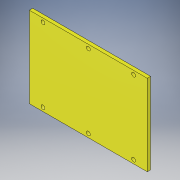
# Autodesk Inventor part: КВ33.000.104 - Крышка
Saved by Autodesk Inventor 2019 (Build 230136000, 136)
## iProperties
Created: 2021-03-13
Part Number: КВ33.000.104 - Крышка
Material: ABS Plastic
Document SubType Name: Modeling
Designer: Петров Иван
Density: 1.06 g/cm^3
Appearance: Yellow
Author: Петров Иван
Autodesk Inventor part; units mm, degrees
ref_plane "YZ Plane" through (0, 0, 0) normal (1, 0, 0) x (0, 1, 0)
ref_plane "XZ Plane" through (0, 0, 0) normal (0, 1, 0) x (-1, 0, 0)
ref_plane "XY Plane" through (0, 0, 0) normal (0, 0, 1) x (1, 0, 0)
sketch "Sketch1" plane through (0, 0, 0) normal (0, 0, 1) x (1, 0, 0)
  circle A0 centre (40, -0.1123) radius 1.75 projected
  circle A1 centre (0, -0.1123) radius 1.75 projected
  circle A2 centre (-40, -0.1123) radius 1.75 projected
  line L0 (-44, 3.3877) -> (44, 3.3877) projected
  line L1 (-44, -3.3877) -> (-44, 3.3877) projected
  line L2 (44, -3.3877) -> (-44, -3.3877) projected
  line L3 (44, 3.3877) -> (44, -3.3877) projected
  circle A3 centre (-40, 64.7863) radius 1.75 projected
  circle A4 centre (0, 64.7863) radius 1.75 projected
  circle A5 centre (40, 64.7863) radius 1.75 projected
  line L4 (44, 61.2863) -> (-44, 61.2863) projected
  line L5 (44, 68.0616) -> (44, 61.2863) projected
  line L6 (-44, 68.0616) -> (44, 68.0616) projected
  line L7 (-44, 61.2863) -> (-44, 68.0616) projected
  line L8 (44, 68.0616) -> (44, -3.3877) projected
  line L9 (44, -3.3877) -> (47, -3.3877) projected
  line L10 (47, 68.0616) -> (47, -3.3877) projected
  line L11 (44, 68.0616) -> (47, 68.0616) projected
  line L12 (-47, 68.0616) -> (-47, -3.3877) projected
  line L13 (-47, -3.3877) -> (-44, -3.3877) projected
  line L14 (-44, 68.0616) -> (-44, -3.3877) projected
  line L15 (-47, 68.0616) -> (-44, 68.0616) projected
  line L16 (-47, -3.3877) -> (-52, -3.3877)
  line L17 (-52, -3.3877) -> (-52, 68.0616)
  line L18 (-52, 68.0616) -> (-47, 68.0616)
  line L19 (-47, 68.0616) -> (-47, -3.3877)
  line L20 (47, -3.3877) -> (52, -3.3877)
  line L21 (52, -3.3877) -> (52, 68.0616)
  line L22 (52, 68.0616) -> (47, 68.0616)
  line L23 (47, 68.0616) -> (47, -3.3877)
  point P0 (0, 0)
  dimension "d0" = 5
  dimension "d1" = 5
  constraints: 16 end point, 4 parallel, 2 horizontal, 2 perpendicular
  measures "d0" distance of L12.start L17.end
  measures "d1" distance of L10.start L21.end
extrude "Extrusion1" add sketch "Sketch1" along normal blind 3
equation "\"BendRadius\" = Thickness"
equation "\"BendReliefWidth\" = Thickness"
equation "\"BendReliefDepth\" = 0.5 * Thickness"
equation "\"CornerReliefSize\" = 4 * Thickness"
equation "\"MinimumRemnant\" = 2 * Thickness"
equation "\"TransitionRadius\" = BendRadius"
equation "\"JacobiRadiusSize\" = Thickness"
equation "\"GapSize\" = Thickness"
equation "\"Thickness\" = 0.5"
body "Solid1"
